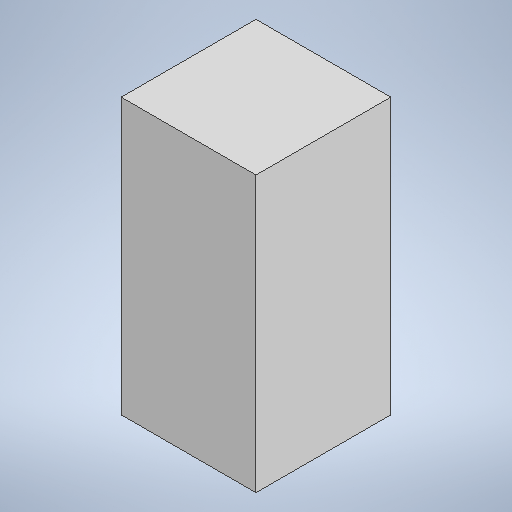
# Autodesk Inventor part: CVTag
Saved by Autodesk Inventor 2025.2 (Build 292293000, 293)
## iProperties
Created: 2025-03-26
Part Number: CVTag
Material: Generic
Document SubType Name: Modeling
Designer: Marcu
Density: 1 g/cm^3
Appearance: Default
Author: Marcu
Autodesk Inventor part; units mm, degrees
ref_plane "YZ Plane" through (0, 0, 0) normal (1, 0, 0) x (0, 1, 0)
ref_plane "XZ Plane" through (0, 0, 0) normal (0, 1, 0) x (-1, 0, 0)
ref_plane "XY Plane" through (0, 0, 0) normal (0, 0, 1) x (1, 0, 0)
sketch "Sketch1" plane through (0, 0, 0) normal (0, 1, 0) x (-1, 0, 0)
  line L0 (-2.45, -2.45) -> (2.45, -2.45)
  line L1 (2.45, -2.45) -> (2.45, 2.45)
  line L2 (2.45, 2.45) -> (-2.45, 2.45)
  line L3 (-2.45, 2.45) -> (-2.45, -2.45)
  point P0 (0, 0)
  dimension "d0" = 2.45
  dimension "d1" = 2.45
  dimension "d2" = 4.9
  dimension "d3" = 4.9
  constraints: 8 end point, 2 parallel, 1 horizontal, 1 perpendicular
  measures "d0" distance from line of point (0, 0) L2
  measures "d1" distance from line of point (0, 0) L1
  measures "d2" distance between parallel lines of L2 L0
  measures "d3" distance between parallel lines of L3 L1
extrude "Extrusion1" add sketch "Sketch1" along normal blind 10
body "Solid1"
